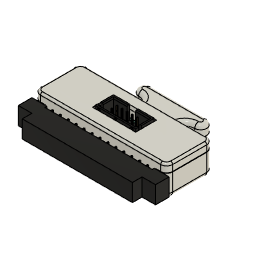
CBM8296_UP_Dongle v2 (Autodesk Fusion 360 design; units mm, degrees)
Autodesk Fusion 360 part; units mm, degrees
sketch "PCB" plane through (0, 0, 0) normal (0, 0, 1) x (1, 0, 0) in component "PCB"
  line L0 (54, 20) -> (0, 20)
  line L1 (0, 0) -> (54, 0)
  line L2 (54, 0) -> (54, 20)
  line L3 (0, 20) -> (0, 0)
  line L4 (1.3215, 4.5593) -> (1.3215, 2.9337)
  line L5 (2.4331, 2.9337) -> (3.3362, 2.9337)
  arc A0 (3.3362, 4.1529) -> (2.9298, 4.5593) centre (2.9298, 4.1529) ccw
  arc A1 (2.9298, 4.5593) -> (2.4331, 4.1981) centre (2.9298, 4.0372) ccw
  line L6 (0.87, 4.1981) -> (1.3215, 4.5593)
  line L7 (0.87, 2.9337) -> (1.7731, 2.9337)
  arc A2 (3.2007, 3.8368) -> (3.3362, 4.1529) centre (2.8997, 4.1529) ccw
  line L8 (3.2007, 3.8368) -> (2.4331, 2.9337)
  line L9 (43.09, -1) -> (43.09, 0)
  line L10 (46.55, 0) -> (46.55, -1)
  line L11 (51.01, -1) -> (51.01, 0)
  line L12 (51.01, 0) -> (50.51, 0)
  circle A3 centre (5, 15) radius 3.1789
  line L13 (50.51, 0) -> (50.51, -1)
  line L14 (45.82, 0.1) -> (45.82, -1)
  line L15 (43.09, 0) -> (42.59, 0)
  circle A4 centre (5, 15) radius 1.7463
  circle A5 centre (49, 15) radius 3.1789
  circle A6 centre (49, 15) radius 1.7463
  line L16 (49.78, 0.1) -> (49.78, -1)
  line L17 (43.82, 0.1) -> (43.82, -1)
  line L18 (7.45, -1) -> (7.45, 0)
  line L19 (3.49, 0) -> (2.99, 0)
  line L20 (37.9, 0.1) -> (37.9, -1)
  line L21 (24.02, 0.1) -> (24.02, -1)
  line L22 (34.67, 0) -> (34.67, -1)
  line L23 (22.79, 0) -> (22.79, -1)
  line L24 (23.29, 0) -> (22.79, 0)
  line L25 (29.98, 0.1) -> (29.98, -1)
  line L26 (38.63, 0) -> (38.63, -1)
  line L27 (35.17, -1) -> (35.17, 0)
  line L28 (27.25, 0) -> (26.75, 0)
  line L29 (26.75, 0) -> (26.75, -1)
  line L30 (35.17, 0) -> (34.67, 0)
  line L31 (47.05, -1) -> (47.05, 0)
  line L32 (33.94, 0.1) -> (33.94, -1)
  line L33 (23.29, -1) -> (23.29, 0)
  line L34 (47.05, 0) -> (46.55, 0)
  line L35 (27.98, 0.1) -> (27.98, -1)
  line L36 (42.59, 0) -> (42.59, -1)
  line L37 (41.86, 0.1) -> (41.86, -1)
  line L38 (35.9, 0.1) -> (35.9, -1)
  line L39 (30.71, 0) -> (30.71, -1)
  line L40 (27.25, -1) -> (27.25, 0)
  line L41 (31.94, 0.1) -> (31.94, -1)
  line L42 (39.86, 0.1) -> (39.86, -1)
  line L43 (26.02, 0.1) -> (26.02, -1)
  line L44 (39.13, 0) -> (38.63, 0)
  line L45 (47.78, 0.1) -> (47.78, -1)
  line L46 (31.21, 0) -> (30.71, 0)
  line L47 (10.18, 0.1) -> (10.18, -1)
  line L48 (7.45, 0) -> (6.95, 0)
  line L49 (8.18, 0.1) -> (8.18, -1)
  line L50 (6.22, 0.1) -> (6.22, -1)
  line L51 (4.22, 0.1) -> (4.22, -1)
  line L52 (3.49, -1) -> (3.49, 0)
  line L53 (39.13, -1) -> (39.13, 0)
  line L54 (31.21, -1) -> (31.21, 0)
  line L55 (53.8, -1) -> (0.2, -1)
  line L56 (6.95, 0) -> (6.95, -1)
  line L57 (0.2, -1) -> (0.2, 0)
  line L58 (0.2, 0) -> (-2.3, 0)
  line L59 (14.14, 0.1) -> (14.14, -1)
  line L60 (2.99, 0) -> (2.99, -1)
  line L61 (-7.25, 0) -> (-7.25, -6.8)
  line L62 (-2.3, 0) -> (-4, 0)
  line L63 (61.25, 0) -> (61.25, -6.8)
  line L64 (58, 0) -> (56.3, 0)
  line L65 (59.7, 0) -> (58, 0)
  line L66 (18.83, 0) -> (18.83, -1)
  line L67 (14.87, 0) -> (14.87, -1)
  line L68 (20.06, 0.1) -> (20.06, -1)
  line L69 (22.06, 0.1) -> (22.06, -1)
  line L70 (19.33, -1) -> (19.33, 0)
  line L71 (56.3, -1.6) -> (56.3, 0)
  line L72 (35.89, 15.3338) -> (35.89, 10.2537)
  line L73 (18.1, 0.1) -> (18.1, -1)
  line L74 (37.16, 8.825) -> (37.16, 7.3962)
  line L75 (16.84, 8.825) -> (16.84, 10.2537)
  line L76 (-4, 0) -> (-5.7, 0)
  line L77 (56.3, -6.8) -> (56.3, -5.2)
  line L78 (-2.3, -1.6) -> (-2.3, 0)
  line L79 (37.16, 7.3962) -> (16.84, 7.3962)
  line L80 (-5.7, -4.2) -> (-5.7, -2.6)
  line L81 (58, -7.2333) -> (58, -4.3667)
  line L82 (16.84, 7.3962) -> (16.84, 8.825)
  line L83 (16.1, 0.1) -> (16.1, -1)
  line L84 (-4, -8.7333) -> (-4, -11.6)
  line L85 (-5.7, -6.8) -> (-7.25, -6.8)
  line L86 (15.37, -1) -> (15.37, 0)
  line L87 (19.33, 0) -> (18.83, 0)
  line L88 (58, -8.052) -> (58, -7.9147)
  line L89 (-2.3, -4.2) -> (-2.3, -2.6)
  line L90 (-5.7, -6.8) -> (-5.7, -5.2)
  line L91 (18.11, 10.2537) -> (18.11, 15.3338)
  line L92 (12.14, 0.1) -> (12.14, -1)
  line L93 (59.7, -1.6) -> (59.7, 0)
  line L94 (15.37, 0) -> (14.87, 0)
  line L95 (29.0638, 16.6038) -> (37.16, 16.6038)
  line L96 (18.11, 15.3338) -> (24.9362, 15.3338)
  line L97 (16.84, 10.2537) -> (16.84, 16.6038)
  line L98 (-2.3, -6.8) -> (-2.3, -5.2)
  line L99 (10.91, 0) -> (10.91, -1)
  line L100 (24.9362, 16.6038) -> (29.0638, 16.6038)
  line L101 (11.41, -1) -> (11.41, 0)
  line L102 (24.9362, 15.3338) -> (29.0638, 15.3338)
  line L103 (56.3, -6.8) -> (54.5, -6.8)
  line L104 (11.41, 0) -> (10.91, 0)
  line L105 (-4, -4.3667) -> (-4, -7.2333)
  line L106 (59.7, -6.8) -> (59.7, -5.2)
  line L107 (37.16, 10.2537) -> (37.16, 8.825)
  line L108 (56.3, -4.2) -> (56.3, -2.6)
  line L109 (16.84, 16.6038) -> (24.9362, 16.6038)
  line L110 (-2.3, -6.8) -> (-5.7, -6.8)
  line L111 (54.5, -11.6) -> (-0.5, -11.6)
  line L112 (35.89, 8.6662) -> (18.11, 8.6662)
  line L113 (29.0638, 15.3338) -> (35.89, 15.3338)
  line L114 (35.89, 8.825) -> (35.89, 8.6662)
  line L115 (58, -2.8667) -> (58, 0)
  line L116 (-4, -3.548) -> (-4, -3.6853)
  line L117 (58, -3.6853) -> (58, -3.548)
  line L118 (-5.7, -1.6) -> (-5.7, 0)
  line L119 (17.6337, 10.2537) -> (16.84, 10.2537)
  line L120 (59.7, -4.2) -> (59.7, -2.6)
  line L121 (-4, -7.9147) -> (-4, -8.052)
  line L122 (58, -11.6) -> (58, -8.7333)
  line L123 (32.08, 14.6987) -> (32.3975, 15.0162)
  line L124 (61.25, 0) -> (59.7, 0)
  line L125 (36.3663, 8.19) -> (17.6337, 8.19)
  line L126 (36.3663, 8.19) -> (35.89, 8.6662)
  line L127 (35.89, 8.825) -> (36.3663, 8.825)
  line L128 (35.89, 10.2537) -> (36.3663, 10.2537)
  arc A7 (26.5238, 7.3962) -> (27.635, 7.3962) centre (27.0794, 7.3962) ccw
  line L129 (18.11, 8.6662) -> (17.6337, 8.19)
  line L130 (59.7, -6.8) -> (56.3, -6.8)
  line L131 (53.8, 0) -> (53.8, -1)
  line L132 (32.715, 15.0162) -> (32.5563, 15.0162)
  line L133 (32.5563, 15.0162) -> (32.3975, 15.0162)
  line L134 (31.9213, 15.0162) -> (32.08, 14.8575)
  line L135 (36.3663, 8.825) -> (37.16, 8.825)
  line L136 (36.3663, 8.19) -> (36.3663, 8.825)
  line L137 (24.9362, 15.3338) -> (24.9362, 15.81)
  line L138 (31.9213, 15.0162) -> (31.7625, 15.0162)
  line L139 (56.3, 0) -> (53.8, 0)
  line L140 (-4, 0) -> (-4, -2.8667)
  line L141 (24.9362, 15.81) -> (24.9362, 16.6038)
  line L142 (31.7625, 15.0162) -> (32.08, 14.6987)
  line L143 (18.11, 10.2537) -> (17.6337, 10.2537)
  line L144 (31.7625, 15.0162) -> (31.6038, 15.0162)
  line L145 (29.0638, 15.81) -> (36.3663, 15.81)
  line L146 (32.08, 14.54) -> (32.5563, 15.0162)
  line L147 (29.0638, 15.3338) -> (29.0638, 15.81)
  line L148 (18.11, 8.825) -> (18.11, 10.2537)
  line L149 (54.5, -6.8) -> (54.5, -11.6)
  line L150 (31.6038, 15.0162) -> (32.08, 14.54)
  line L151 (31.445, 15.0162) -> (32.08, 14.3812)
  line L152 (36.3663, 15.81) -> (35.89, 15.3338)
  line L153 (35.89, 10.2537) -> (35.89, 8.825)
  line L154 (-5.7, 0) -> (-7.25, 0)
  line L155 (18.11, 15.3338) -> (17.6337, 15.81)
  line L156 (-0.5, -11.6) -> (-0.5, -6.8)
  line L157 (17.6337, 8.825) -> (16.84, 8.825)
  arc A8 (18.11, 7.3962) -> (19.38, 7.3962) centre (18.745, 7.3962) ccw
  arc A9 (34.62, 7.3962) -> (35.89, 7.3962) centre (35.255, 7.3962) ccw
  line L158 (29.0638, 15.81) -> (29.0638, 16.6038)
  line L159 (-0.5, -6.8) -> (-2.3, -6.8)
  line L160 (32.08, 14.8575) -> (32.2388, 15.0162)
  line L161 (32.2388, 15.0162) -> (31.9213, 15.0162)
  line L162 (61.25, -6.8) -> (59.7, -6.8)
  line L163 (18.11, 8.6662) -> (18.11, 8.825)
  line L164 (37.16, 16.6038) -> (37.16, 10.2537)
  line L165 (31.6038, 15.0162) -> (31.445, 15.0162)
  line L166 (17.6337, 10.2537) -> (17.6337, 15.81)
  line L167 (32.08, 14.3812) -> (32.715, 15.0162)
  line L168 (32.3975, 15.0162) -> (32.2388, 15.0162)
  line L169 (36.3663, 10.2537) -> (36.3663, 15.81)
  line L170 (18.11, 8.825) -> (17.6337, 8.825)
  line L171 (36.3663, 10.2537) -> (37.16, 10.2537)
  line L172 (24.9362, 15.81) -> (17.6337, 15.81)
  line L173 (17.6337, 8.825) -> (17.6337, 8.19)
  line L174 (49.78, 0.1) -> (49.78, 4)
  line L175 (49.28, 3) -> (49.28, 2)
  arc A10 (44.32, 2) -> (45.32, 2) centre (44.82, 2) ccw
  line L176 (45.82, 0.1) -> (45.82, 4)
  line L177 (45.32, 3) -> (45.32, 2)
  arc A11 (45.32, 3) -> (44.32, 3) centre (44.82, 3) ccw
  arc A12 (49.78, 4) -> (47.78, 4) centre (48.78, 4) ccw
  arc A13 (49.28, 3) -> (48.28, 3) centre (48.78, 3) ccw
  line L178 (47.78, 0.1) -> (47.78, 4)
  arc A14 (45.82, 4) -> (43.82, 4) centre (44.82, 4) ccw
  line L179 (44.32, 3) -> (44.32, 2)
  line L180 (20.56, 3) -> (20.56, 2)
  arc A15 (17.6, 3) -> (16.6, 3) centre (17.1, 3) ccw
  line L181 (41.86, 0.1) -> (41.86, 4)
  arc A16 (33.44, 3) -> (32.44, 3) centre (32.94, 3) ccw
  line L182 (13.64, 3) -> (13.64, 2)
  arc A17 (6.22, 4) -> (4.22, 4) centre (5.22, 4) ccw
  line L183 (12.14, 0.1) -> (12.14, 4)
  arc A18 (5.72, 3) -> (4.72, 3) centre (5.22, 3) ccw
  arc A19 (26.02, 4) -> (24.02, 4) centre (25.02, 4) ccw
  arc A20 (36.4, 2) -> (37.4, 2) centre (36.9, 2) ccw
  arc A21 (48.28, 2) -> (49.28, 2) centre (48.78, 2) ccw
  arc A22 (24.52, 2) -> (25.52, 2) centre (25.02, 2) ccw
  line L184 (39.86, 0.1) -> (39.86, 4)
  arc A23 (28.48, 2) -> (29.48, 2) centre (28.98, 2) ccw
  arc A24 (16.6, 2) -> (17.6, 2) centre (17.1, 2) ccw
  arc A25 (10.18, 4) -> (8.18, 4) centre (9.18, 4) ccw
  line L185 (24.52, 3) -> (24.52, 2)
  arc A26 (18.1, 4) -> (16.1, 4) centre (17.1, 4) ccw
  arc A27 (13.64, 3) -> (12.64, 3) centre (13.14, 3) ccw
  arc A28 (9.68, 3) -> (8.68, 3) centre (9.18, 3) ccw
  arc A29 (33.94, 4) -> (31.94, 4) centre (32.94, 4) ccw
  arc A30 (41.86, 4) -> (39.86, 4) centre (40.86, 4) ccw
  line L186 (33.94, 0.1) -> (33.94, 4)
  arc A31 (20.56, 2) -> (21.56, 2) centre (21.06, 2) ccw
  line L187 (35.9, 0.1) -> (35.9, 4)
  line L188 (29.98, 0.1) -> (29.98, 4)
  line L189 (33.44, 3) -> (33.44, 2)
  line L190 (41.36, 3) -> (41.36, 2)
  arc A32 (4.72, 2) -> (5.72, 2) centre (5.22, 2) ccw
  line L191 (5.72, 3) -> (5.72, 2)
  line L192 (9.68, 3) -> (9.68, 2)
  line L193 (21.56, 3) -> (21.56, 2)
  line L194 (36.4, 3) -> (36.4, 2)
  line L195 (12.64, 3) -> (12.64, 2)
  line L196 (4.22, 0.1) -> (4.22, 4)
  line L197 (48.28, 3) -> (48.28, 2)
  arc A33 (8.68, 2) -> (9.68, 2) centre (9.18, 2) ccw
  line L198 (17.6, 3) -> (17.6, 2)
  arc A34 (22.06, 4) -> (20.06, 4) centre (21.06, 4) ccw
  arc A35 (41.36, 3) -> (40.36, 3) centre (40.86, 3) ccw
  line L199 (37.9, 0.1) -> (37.9, 4)
  line L200 (32.44, 3) -> (32.44, 2)
  line L201 (31.94, 0.1) -> (31.94, 4)
  line L202 (4.72, 3) -> (4.72, 2)
  arc A36 (37.4, 3) -> (36.4, 3) centre (36.9, 3) ccw
  arc A37 (29.48, 3) -> (28.48, 3) centre (28.98, 3) ccw
  line L203 (16.6, 3) -> (16.6, 2)
  line L204 (20.06, 0.1) -> (20.06, 4)
  arc A38 (40.36, 2) -> (41.36, 2) centre (40.86, 2) ccw
  line L205 (27.98, 0.1) -> (27.98, 4)
  line L206 (26.02, 0.1) -> (26.02, 4)
  line L207 (24.02, 0.1) -> (24.02, 4)
  line L208 (28.48, 3) -> (28.48, 2)
  arc A39 (29.98, 4) -> (27.98, 4) centre (28.98, 4) ccw
  arc A40 (37.9, 4) -> (35.9, 4) centre (36.9, 4) ccw
  line L209 (29.48, 3) -> (29.48, 2)
  line L210 (6.22, 0.1) -> (6.22, 4)
  line L211 (43.82, 0.1) -> (43.82, 4)
  arc A41 (25.52, 3) -> (24.52, 3) centre (25.02, 3) ccw
  arc A42 (32.44, 2) -> (33.44, 2) centre (32.94, 2) ccw
  line L212 (25.52, 3) -> (25.52, 2)
  line L213 (22.06, 0.1) -> (22.06, 4)
  line L214 (37.4, 3) -> (37.4, 2)
  line L215 (40.36, 3) -> (40.36, 2)
  line L216 (24.206, 13.016) -> (24.714, 13.016)
  line L217 (31.826, 10.984) -> (31.826, 10.476)
  line L218 (31.826, 10.476) -> (32.334, 10.476)
  line L219 (31.826, 13.016) -> (32.334, 13.016)
  line L220 (32.334, 13.016) -> (32.334, 13.524)
  line L221 (24.714, 13.524) -> (24.206, 13.524)
  line L222 (29.286, 10.476) -> (29.794, 10.476)
  line L223 (29.286, 13.524) -> (29.286, 13.016)
  line L224 (31.826, 13.524) -> (31.826, 13.016)
  line L225 (24.206, 10.984) -> (24.206, 10.476)
  line L226 (26.746, 10.476) -> (27.254, 10.476)
  line L227 (26.746, 13.524) -> (26.746, 13.016)
  line L228 (29.794, 10.984) -> (29.286, 10.984)
  line L229 (14.14, 0.1) -> (14.14, 4)
  line L230 (21.666, 13.016) -> (22.174, 13.016)
  line L231 (21.666, 13.524) -> (21.666, 13.016)
  line L232 (21.666, 10.476) -> (22.174, 10.476)
  line L233 (8.18, 0.1) -> (8.18, 4)
  line L234 (22.174, 13.016) -> (22.174, 13.524)
  line L235 (27.254, 10.476) -> (27.254, 10.984)
  line L236 (29.794, 13.524) -> (29.286, 13.524)
  line L237 (24.714, 10.984) -> (24.206, 10.984)
  line L238 (24.206, 13.524) -> (24.206, 13.016)
  line L239 (29.794, 13.016) -> (29.794, 13.524)
  line L240 (10.18, 0.1) -> (10.18, 4)
  line L241 (16.1, 0.1) -> (16.1, 4)
  line L242 (32.334, 10.984) -> (31.826, 10.984)
  line L243 (29.286, 10.984) -> (29.286, 10.476)
  arc A43 (12.64, 2) -> (13.64, 2) centre (13.14, 2) ccw
  line L244 (29.794, 10.476) -> (29.794, 10.984)
  line L245 (29.286, 13.016) -> (29.794, 13.016)
  line L246 (8.68, 3) -> (8.68, 2)
  line L247 (32.334, 13.524) -> (31.826, 13.524)
  line L248 (24.714, 13.016) -> (24.714, 13.524)
  arc A44 (14.14, 4) -> (12.14, 4) centre (13.14, 4) ccw
  line L249 (27.254, 10.984) -> (26.746, 10.984)
  line L250 (24.206, 10.476) -> (24.714, 10.476)
  line L251 (18.1, 0.1) -> (18.1, 4)
  line L252 (44, 12.25) -> (44, 12.2)
  line L253 (26.746, 13.016) -> (27.254, 13.016)
  line L254 (22.174, 10.984) -> (21.666, 10.984)
  line L255 (21.666, 10.984) -> (21.666, 10.476)
  line L256 (26.746, 10.984) -> (26.746, 10.476)
  line L257 (22.174, 10.476) -> (22.174, 10.984)
  line L258 (24.714, 10.476) -> (24.714, 10.984)
  line L259 (27.254, 13.524) -> (26.746, 13.524)
  line L260 (32.334, 10.476) -> (32.334, 10.984)
  arc A45 (21.56, 3) -> (20.56, 3) centre (21.06, 3) ccw
  line L261 (27.254, 13.016) -> (27.254, 13.524)
  line L262 (22.174, 13.524) -> (21.666, 13.524)
extrude "Extrude1" add sketch "PCB" against normal blind 1.6 contours L0 L1 L2 L3 L12 L14 L15 L16 L17 L19 L20 L21 L24 L25 L28 L30 L32 L34 L35 L37 L38 L41 L42 L43 L44 L45 L46 L47 L48 L49 L50 L51 L58 L59 L68 L69 L73 L83 L87 L92 L94 L104 L139 L174 L176 A12 L178 A14 L181 A17 L183 A19 L184 A25 A26 A29 A30 L186 L187 L188 L196 A34 L199 L201 L204 L205 L206 L207 A39 A40 L210 L211 L213 L229 L233 L240 L241 A44 L251 | L1 L16 L45 L174 A12 L178 | L1 L50 L51 A17 L196 L210 | L1 L14 L17 L176 A14 L211 | L1 L47 L49 A25 L233 L240 | L1 L37 L42 L181 L184 A30 | L1 L59 L92 L183 L229 A44 | L1 L20 L38 L187 L199 A40 | L1 L73 L83 A26 L241 L251 | L1 L32 L41 A29 L186 L201 | L1 L68 L69 A34 L204 L213 | L1 L25 L35 L188 L205 A39 | L1 L21 L43 A19 L206 L207 | A3 | A5 | L72 L128 L152 L169 | L72 L91 L96 L102 L112 L113 L114 L148 L153 L163 | L113 L145 L147 L152 | L107 L127 L128 L135 L153 L171 | L100 L102 L137 L141 L147 L158 | L95 L145 L158 L164 L169 L171 | L114 L126 L127 L136 | L96 L137 L155 L172 | L112 L125 L126 L129 | L74 L79 L82 L125 L135 L136 L157 L173 | L91 L143 L155 L166 | L97 L109 L119 L141 L166 L172 | L129 L163 L170 L173 | L75 L119 L143 L148 L157 L170 | L79 A9 | L79 A7 | L79 A8 | L123 L134 L138 L142 L160 L168 | L123 L133 L142 L144 L146 L150 | L132 L146 L150 L151 L165 L167 | L134 L160 L161 | L175 A13 A21 L197 | A10 L177 A11 L179 | L180 A31 L193 A45 | A15 A24 L198 L203 | A16 L189 L200 A42 | L182 A27 L195 A43 | A18 A32 L191 L202 | A20 L194 A36 L214 | A22 L185 A41 L212 | A23 A37 L208 L209 | A28 L192 A33 L246 | L190 A35 A38 L215 | L216 L221 L238 L248 | L217 L218 L242 L260 | L219 L220 L224 L247 | L222 L228 L243 L244 | L223 L236 L239 L245 | L225 L237 L250 L258 | L226 L235 L249 L256 | L227 L253 L259 L261 | L230 L231 L234 L262 | L232 L254 L255 L257 makes body 1 in component "PCB"
extrude "Extrude5" add sketch "PCB" along normal blind 2.3 contours L72 L91 L96 L102 L112 L113 L114 L148 L153 L163 | L107 L127 L128 L135 L153 L171 | L100 L102 L137 L141 L147 L158 | L75 L119 L143 L148 L157 L170 bodies 1 in component "PCB"
extrude "Extrude6" add sketch "PCB" along normal blind 9.3 contours L72 L128 L152 L169 | L113 L145 L147 L152 | L95 L145 L158 L164 L169 L171 | L114 L126 L127 L136 | L96 L137 L155 L172 | L112 L125 L126 L129 | L74 L79 L82 L125 L135 L136 L157 L173 | L91 L143 L155 L166 | L97 L109 L119 L141 L166 L172 | L129 L163 L170 L173 bodies 1 in component "PCB"
extrude "Extrude7" add sketch "PCB" along normal blind 8.8 contours L216 L221 L238 L248 | L217 L218 L242 L260 | L219 L220 L224 L247 | L222 L228 L243 L244 | L223 L236 L239 L245 | L225 L237 L250 L258 | L226 L235 L249 L256 | L227 L253 L259 L261 | L230 L231 L234 L262 | L232 L254 L255 L257 bodies 1 in component "PCB"
extrude "Extrude8" add sketch "PCB" along normal blind 8.8 contours L79 A9 | L79 A7 | L79 A8 bodies 1 in component "PCB"
extrude "Extrude9" add sketch "PCB" along normal blind 4.3 and the other way blind 4.4 contours L1 L55 L57 L58 L61 L62 L63 L64 L65 L76 L85 L103 L110 L111 L124 L130 L131 L139 L149 L154 L156 L159 L162 | L1 L11 L12 L13 L55 | L1 L19 L52 L55 L60 | L1 L10 L31 L34 L55 | L1 L18 L48 L55 L56 | L1 L9 L15 L36 L55 | L1 L55 L99 L101 L104 | L1 L26 L44 L53 L55 | L1 L55 L67 L86 L94 | L1 L22 L27 L30 L55 | L1 L55 L66 L70 L87 | L1 L39 L46 L54 L55 | L1 L23 L24 L33 L55 | L1 L28 L29 L40 L55 bodies 1 in component "PCB"
extrude "Extrude10" add sketch "PCB" along normal blind 0.5 contours L1 L16 L45 L55 | L1 L16 L45 L174 A12 L178 | L1 L50 L51 A17 L196 L210 | L1 L50 L51 L55 | L1 L14 L17 L55 | L1 L14 L17 L176 A14 L211 | L1 L47 L49 A25 L233 L240 | L1 L47 L49 L55 | L1 L37 L42 L55 | L1 L37 L42 L181 L184 A30 | L1 L59 L92 L183 L229 A44 | L1 L55 L59 L92 | L1 L20 L38 L55 | L1 L20 L38 L187 L199 A40 | L1 L73 L83 A26 L241 L251 | L1 L55 L73 L83 | L1 L32 L41 L55 | L1 L32 L41 A29 L186 L201 | L1 L68 L69 A34 L204 L213 | L1 L55 L68 L69 | L1 L25 L35 L55 | L1 L25 L35 L188 L205 A39 | L1 L21 L43 A19 L206 L207 | L1 L21 L43 L55 bodies 1 in component "PCB"
extrude "Extrude11" add sketch "PCB" against normal blind 0.5 from surface at -1.6 contours L1 L16 L45 L55 | L1 L16 L45 L174 A12 L178 | L1 L50 L51 A17 L196 L210 | L1 L50 L51 L55 | L1 L14 L17 L55 | L1 L14 L17 L176 A14 L211 | L1 L47 L49 A25 L233 L240 | L1 L47 L49 L55 | L1 L37 L42 L55 | L1 L37 L42 L181 L184 A30 | L1 L59 L92 L183 L229 A44 | L1 L55 L59 L92 | L1 L20 L38 L55 | L1 L20 L38 L187 L199 A40 | L1 L73 L83 A26 L241 L251 | L1 L55 L73 L83 | L1 L32 L41 L55 | L1 L32 L41 A29 L186 L201 | L1 L68 L69 A34 L204 L213 | L1 L55 L68 L69 | L1 L25 L35 L55 | L1 L25 L35 L188 L205 A39 | L1 L21 L43 A19 L206 L207 | L1 L21 L43 L55 bodies 1 in component "PCB"
chamfer "Chamfer1" distance 0.5 angle 45 7 edges at (27, 8.6662, 9.3) (35.89, 12.7938, 9.3) (32.4769, 15.3338, 9.3) (21.5231, 15.3338, 9.3) (18.11, 12.7938, 9.3) (18.11, 8.7456, 9.3) (35.89, 8.7456, 9.3) on bodies 1 in component "PCB"
ref_plane "WorkPlane1" through (0, 0, -4.4) normal (0, 0, 1) x (1, 0, 0) in component "bottom_shell"
sketch "bottom" plane through (0, 0, -4.4) normal (0, 0, 1) x (1, 0, 0) in component "bottom_shell"
  circle A0 centre (49, 15) radius 1.7463 construction
  line L0 (54, 0) -> (54, 20) construction
  line L1 (54, 20) -> (0, 20) construction
  line L2 (0, 20) -> (0, 0) construction
  circle A1 centre (5, 15) radius 1.7463 construction
  line L3 (27, 20) -> (27, -5) construction
  line L4 (54, 0) -> (0, 0) construction
  circle A2 centre (49, 15) radius 1.75
  circle A3 centre (5, 15) radius 1.75
  line L5 (60, 3) -> (60, 20)
  line L6 (-6, 3) -> (-6, 20)
  line L7 (57, 23) -> (-3, 23)
  line L8 (57, 0) -> (-3, 0)
  arc A4 (57, 0) -> (60, 3) centre (57, 3) ccw
  arc A5 (60, 20) -> (57, 23) centre (57, 20) ccw
  arc A6 (-3, 23) -> (-6, 20) centre (-3, 20) ccw
  arc A7 (-6, 3) -> (-3, 0) centre (-3, 3) ccw
  line L9 (57, 21) -> (-3, 21)
  arc A8 (-3, 21) -> (-4, 20) centre (-3, 20) ccw
  line L10 (-4, 3) -> (-4, 20)
  arc A9 (-4, 3) -> (-3, 2) centre (-3, 3) ccw
  line L11 (57, 2) -> (-3, 2)
  arc A10 (57, 2) -> (58, 3) centre (57, 3) ccw
  line L12 (58, 3) -> (58, 20)
  arc A11 (58, 20) -> (57, 21) centre (57, 20) ccw
  circle A12 centre (49, 15) radius 4.25
  circle A13 centre (5, 15) radius 4.25
  line L13 (54.6, 1.2) -> (54.6, 2)
  line L14 (-0.6, 0) -> (-0.6, 2)
  circle A14 centre (49, 15) radius 3
  circle A15 centre (5, 15) radius 3
  line L15 (57, 21.8) -> (-3, 21.8)
  arc A16 (-3, 21.8) -> (-4.8, 20) centre (-3, 20) ccw
  line L16 (-4.8, 3) -> (-4.8, 20)
  arc A17 (-4.8, 3) -> (-3, 1.2) centre (-3, 3) ccw
  arc A18 (57, 1.2) -> (58.8, 3) centre (57, 3) ccw
  line L17 (58.8, 3) -> (58.8, 20)
  arc A19 (58.8, 20) -> (57, 21.8) centre (57, 20) ccw
  line L18 (57, 1.2) -> (54.6, 1.2)
  line L19 (-0.6, 1.2) -> (-3, 1.2)
  line L20 (54.6, 1.2) -> (54.6, 0)
  line L21 (41, 28) -> (41, 33) construction
  line L22 (41, 33) -> (13, 33) construction
  line L23 (41, 33) -> (41, 39.5) construction
  line L24 (13, 39) -> (41, 39)
  line L25 (13, 36) -> (13, 39) construction
  arc A20 (13, 39) -> (13, 33) centre (13, 36) ccw
  arc A21 (41, 33) -> (41, 39) centre (41, 36) ccw
  arc A22 (41, 33) -> (41, 23) centre (41, 28) ccw
  arc A23 (13, 23) -> (13, 33) centre (13, 28) ccw
  point P0 (51.01, 0)
  point P1 (60, 0)
  point P2 (60, 23)
  point P3 (-6, 0)
  point P4 (-6, 23)
  dimension "d181" = 3.5
  dimension "d182" = 3.5
  dimension "d186" = 3
  dimension "d187" = 23
  dimension "d188" = 66
  dimension "d190" = 8.5
  dimension "d191" = 8.5
  dimension "d192" = 0.6
  dimension "d193" = 0.6
  dimension "d194" = 6
  dimension "d195" = 6
  dimension "d197" = 1.2
  dimension "d236" = 10
  dimension "d237" = 14
  dimension "d238" = 5
  dimension "d239" = 6
  constraint midpoint L1 L3.start
  constraint perpendicular L1 L3
  constraint coincident L0.start L4.start
  constraint coincident L2.end L4.end
  constraint concentric A0 A2
  constraint concentric A1 A3
  constraint vertical L5
  constraint perpendicular L4 L6
  constraint symmetric L3 L5 L6
  constraint perpendicular L5 L7
  constraint collinear L4 L8
  constraint coincident P1 L5
  constraint tangent L5 A4
  constraint tangent L8 A4
  constraint coincident P2 L5
  constraint coincident P2 L7
  constraint tangent L5 A5
  constraint tangent L7 A5
  constraint equal A4 A5
  constraint coincident P4 L6
  constraint coincident P4 L7
  constraint tangent L6 A6
  constraint tangent L7 A6
  constraint equal A4 A6
  constraint coincident P3 L6
  constraint coincident P3 L8
  constraint tangent L6 A7
  constraint tangent L8 A7
  constraint equal A4 A7
  constraint concentric A0 A12
  constraint concentric A3 A13
  constraint coincident L11 L13.end
  constraint perpendicular L11 L13
  constraint coincident L8 L14.start
  constraint coincident L11 L14.end
  constraint perpendicular L11 L14
  constraint concentric A2 A14
  constraint concentric A3 A15
  constraint parallel L7 L15
  constraint concentric A6 A16
  constraint parallel L6 L16
  constraint concentric A7 A17
  constraint parallel L8 L18
  constraint concentric A4 A18
  constraint parallel L5 L17
  constraint concentric A5 A19
  constraint tangent L15 A19
  constraint tangent A16 L16
  constraint tangent L15 A16
  constraint tangent L17 A19
  constraint tangent L16 A17
  constraint tangent A17 L18
  constraint tangent A18 L18
  constraint tangent A18 L17
  constraint collinear L18 L19
  constraint coincident L14 L19.start
  constraint coincident L8 L20.end
  constraint perpendicular L8 L20
  constraint symmetric L3 A22 A23
  constraint coincident L21.start A22.centre
  constraint vertical L21
  constraint tangent L22 A23
  constraint tangent L22 A21
  constraint perpendicular L22 L23
  constraint coincident A21.centre L23
  constraint symmetric L3 A20 A21
  constraint coincident L23 L24.end
  constraint tangent L24 A21
  constraint coincident L25.start A20.centre
  constraint perpendicular L24 L25
  constraint coincident L7 A22.end
  constraint coincident L7 A23.start
  measures "d181" diameter of A2
  measures "d182" diameter of A3
  measures "d186" radius of A4
  measures "d187" distance of L7 L8
  measures "d188" distance of L5 L6
  measures "d190" diameter of A12
  measures "d191" diameter of A13
  measures "d192" distance of L0 L13
  measures "d193" distance of L2 L14
  measures "d194" diameter of A14
  measures "d195" diameter of A15
  measures "d197" distance of L7 L15
  measures "d236" diameter of A22
  measures "d237" distance of L3 L21.start
  measures "d238" distance of L7 L21.start
  measures "d239" diameter of A21
extrude "Extrude1'" add sketch "bottom" against normal blind 2 separate body contours L5 L6 L7 L8 A4 A5 A6 A7 L14 L15 A16 L16 A17 A18 L17 A19 L18 L19 L20 | L8 L11 L13 L14 L20 | L7 L24 A20 A21 A22 A23 | L9 A8 L10 A9 L11 A10 L12 A11 L13 L14 L15 A16 L16 A17 A18 L17 A19 L18 L19 | L9 A8 L10 A9 L11 A10 L12 A11 | A12 | A13 makes body 2 in component "bottom_shell"
extrude "Extrude2" add sketch "bottom" along normal blind 2.8 contours A12 | A13 | A14 | A15 bodies 2 in component "bottom_shell"
extrude "Extrude3" add sketch "bottom" along normal blind 1.8 contours L8 L11 L13 L14 L20 bodies 2 in component "bottom_shell"
extrude "Extrude4" add sketch "bottom" along normal blind 9.7 contours L9 A8 L10 A9 L11 A10 L12 A11 L13 L14 L15 A16 L16 A17 A18 L17 A19 L18 L19 bodies 2 in component "bottom_shell"
extrude "Extrude5'" add sketch "bottom" along normal blind 8.7 contours L5 L6 L7 L8 A4 A5 A6 A7 L14 L15 A16 L16 A17 A18 L17 A19 L18 L19 L20 bodies 2 in component "bottom_shell"
extrude "Extrude6'" add sketch "bottom" along normal blind 5 contours L7 L24 A20 A21 A22 A23 bodies 2 in component "bottom_shell"
fillet "Fillet1" radius 1 8 edges at (27, 2, -4.4) (57.7071, 2.2929, -4.4) (58, 11.5, -4.4) (57.7071, 20.7071, -4.4) (27, 21, -4.4) (-3.7071, 20.7071, -4.4) (-4, 11.5, -4.4) (-3.7071, 2.2929, -4.4) on bodies 2 in component "bottom_shell"
fillet "Fillet2" radius 1 2 edges at (1.0376, 16.5369, -4.4) (45.0376, 16.5369, -4.4) on bodies 2 in component "bottom_shell"
chamfer "Chamfer1'" distance 1 angle 45 2 edges at (1.0376, 13.4631, -1.6) (45.0376, 13.4631, -1.6) on bodies 2 in component "bottom_shell"
fillet "Fillet4" radius 2 20 edges at (5, 23, -6.4) (18, 28, -6.4) (10, 36, -6.4) (27, 39, -6.4) (44, 36, -6.4) (36, 28, -6.4) (49, 23, -6.4) (59.1213, 22.1213, -6.4) (60, 11.5, -6.4) (59.1213, 0.8787, -6.4) (27, 0, -6.4) (-5.1213, 0.8787, -6.4) (-6, 11.5, -6.4) (-5.1213, 22.1213, -6.4) (36, 28, 0.6) (44, 36, 0.6) (27, 39, 0.6) (10, 36, 0.6) (18, 28, 0.6) (27, 23, 0.6) on bodies 2 in component "bottom_shell"
ref_plane "WorkPlane1" through (0, 0, 6.5) normal (0, 0, 1) x (1, 0, 0) in component "top_shell"
sketch "top" plane through (0, 0, 6.5) normal (0, 0, 1) x (1, 0, 0) in component "top_shell"
  line L0 (16.84, 16.6038) -> (24.9362, 16.6038) construction
  line L1 (24.9362, 16.6038) -> (29.0638, 16.6038) construction
  line L2 (16.84, 10.2537) -> (16.84, 16.6038) construction
  line L3 (16.84, 8.825) -> (16.84, 10.2537) construction
  line L4 (16.84, 7.3962) -> (16.84, 8.825) construction
  line L5 (37.16, 7.3962) -> (16.84, 7.3962) construction
  line L6 (37.16, 8.825) -> (37.16, 7.3962) construction
  line L7 (37.16, 10.2537) -> (37.16, 8.825) construction
  line L8 (37.16, 16.6038) -> (37.16, 10.2537) construction
  line L9 (29.0638, 16.6038) -> (37.16, 16.6038) construction
  line L10 (57, 23) -> (-3, 23)
  arc A0 (-3, 23) -> (-6, 20) centre (-3, 20) ccw
  line L11 (-6, 3) -> (-6, 20)
  arc A1 (-6, 3) -> (-3, 0) centre (-3, 3) ccw
  line L12 (57, 0) -> (-3, 0)
  line L13 (57, 2) -> (-3, 2)
  arc A2 (-4, 3) -> (-3, 2) centre (-3, 3) ccw
  line L14 (-4, 3) -> (-4, 20)
  arc A3 (-3, 21) -> (-4, 20) centre (-3, 20) ccw
  line L15 (57, 21) -> (-3, 21)
  line L16 (58, 3) -> (58, 20)
  arc A4 (58, 20) -> (57, 21) centre (57, 20) ccw
  arc A5 (57, 2) -> (58, 3) centre (57, 3) ccw
  arc A6 (57, 0) -> (60, 3) centre (57, 3) ccw
  line L17 (60, 3) -> (60, 20)
  arc A7 (60, 20) -> (57, 23) centre (57, 20) ccw
  line L18 (-0.6, 0) -> (-0.6, 2)
  line L19 (54.6, 1.2) -> (54.6, 0)
  line L20 (54.6, 1.2) -> (54.6, 2)
  circle A8 centre (5, 15) radius 1.75 construction
  circle A9 centre (49, 15) radius 1.75 construction
  circle A10 centre (5, 15) radius 1.25
  circle A11 centre (49, 15) radius 1.25
  line L21 (16.24, 17.2038) -> (37.76, 17.2038)
  line L22 (37.76, 17.2038) -> (37.76, 6.7962)
  line L23 (37.76, 6.7962) -> (16.24, 6.7962)
  line L24 (16.24, 6.7962) -> (16.24, 17.2038)
  circle A12 centre (5, 15) radius 3.5
  circle A13 centre (49, 15) radius 3.5
  line L25 (59.2, 3) -> (59.2, 20)
  arc A14 (59.2, 20) -> (57, 22.2) centre (57, 20) ccw
  line L26 (57, 22.2) -> (-3, 22.2)
  arc A15 (-3, 22.2) -> (-5.2, 20) centre (-3, 20) ccw
  line L27 (-5.2, 3) -> (-5.2, 20)
  arc A16 (-5.2, 3) -> (-3, 0.8) centre (-3, 3) ccw
  arc A17 (57, 0.8) -> (59.2, 3) centre (57, 3) ccw
  line L28 (57, 0.8) -> (54.6, 0.8)
  line L29 (-0.6, 0.8) -> (-3, 0.8)
  dimension "d213" = 2.5
  dimension "d214" = 2.5
  dimension "d216" = 0.6
  dimension "d217" = 0.6
  dimension "d218" = 0.6
  dimension "d219" = 0.6
  dimension "d220" = 7
  dimension "d221" = 7
  dimension "d223" = 0.8
  constraint concentric A8 A10
  constraint concentric A9 A11
  constraint horizontal L21
  constraint vertical L22
  constraint horizontal L23
  constraint vertical L24
  constraint concentric A10 A12
  constraint concentric A11 A13
  constraint parallel L17 L25
  constraint concentric A7 A14
  constraint parallel L10 L26
  constraint concentric A0 A15
  constraint parallel L11 L27
  constraint concentric A1 A16
  constraint parallel L12 L28
  constraint concentric A6 A17
  constraint tangent L27 A16
  constraint tangent L25 A17
  constraint tangent A16 L28
  constraint tangent L25 A14
  constraint tangent A14 L26
  constraint tangent L26 A15
  constraint tangent A15 L27
  constraint tangent A17 L28
  constraint coincident L19 L28.end
  constraint coincident L18 L29.start
  constraint collinear L28 L29
  measures "d213" diameter of A10
  measures "d214" diameter of A11
  measures "d216" distance of L0 L21
  measures "d217" distance of L5 L23
  measures "d218" distance of L2 L24
  measures "d219" distance of L6 L22
  measures "d220" diameter of A12
  measures "d221" diameter of A13
  measures "d223" distance of L10 L26
extrude "Extrude1''" add sketch "top" along normal blind 2 separate body contours L10 A0 L11 A1 L12 A6 L17 A7 L18 L19 L25 A14 L26 A15 L27 A16 A17 L28 L29 | L12 L13 L18 L19 L20 | L13 A2 L14 A3 L15 L16 A4 A5 L18 L19 L20 L25 A14 L26 A15 L27 A16 A17 L28 L29 | L13 A2 L14 A3 L15 L16 A4 A5 | A10 | A11 | A12 | A13 makes body 3 in component "top_shell"
extrude "Extrude2'" add sketch "top" against normal blind 6.3 contours A12 | A13 bodies 3 in component "top_shell"
extrude "Extrude3'" add sketch "top" against normal blind 1 contours L13 A2 L14 A3 L15 L16 A4 A5 L18 L19 L20 L25 A14 L26 A15 L27 A16 A17 L28 L29 bodies 3 in component "top_shell"
extrude "Extrude4'" add sketch "top" against normal blind 3.5 contours L12 L13 L18 L19 L20 bodies 3 in component "top_shell"
extrude "Extrude5''" add sketch "top" against normal blind 2 contours L10 A0 L11 A1 L12 A6 L17 A7 L18 L19 L25 A14 L26 A15 L27 A16 A17 L28 L29 bodies 3 in component "top_shell"
fillet "Fillet1'" radius 1 10 edges at (27, 21, 6.5) (57.7071, 20.7071, 6.5) (58, 11.5, 6.5) (57.7071, 2.2929, 6.5) (27, 2, 6.5) (-3.7071, 2.2929, 6.5) (-4, 11.5, 6.5) (-3.7071, 20.7071, 6.5) (1.7369, 13.7343, 6.5) (45.7369, 13.7343, 6.5) on bodies 3 in component "top_shell"
fillet "Fillet2'" radius 1 8 edges at (-6, 11.5, 8.5) (-5.1213, 0.8787, 8.5) (27, 0, 8.5) (59.1213, 0.8787, 8.5) (60, 11.5, 8.5) (59.1213, 22.1213, 8.5) (27, 23, 8.5) (-5.1213, 22.1213, 8.5) on bodies 3 in component "top_shell"
component "PCB" placed x (1, 0, 0) y (0, 1, 0) z (0, 0, 1) at (0, 0, 0)
component "bottom_shell" placed x (1, 0, 0) y (0, 1, 0) z (0, 0, 1) at (0, 0, 0)
component "top_shell" placed x (1, 0, 0) y (0, 1, 0) z (0, 0, 1) at (0, 0, 0)
equation "pcb_thickness = 1.6 mm"
equation "below = 2.8 mm + pcb_thickness"
equation "wall = 2 mm"
equation "width = pcb_width + 2 mm + 2 * r_corner + 2 * wall"
equation "length = pcb_length + 1 mm + wall"
equation "above = 8.5 mm - wall"
equation "pcb_width = 54 mm"
equation "pcb_length = 20 mm"
equation "r_corner = 3 mm"
equation "drill = 3.5 mm"
equation "d_screw = 7 mm"
equation "tol_x = 0.3 mm"
equation "tol_connector = 0.6 mm"
equation "d_post = 8.5 mm"
equation "d_post2 = 8 mm"
equation "bottom_height = 4.3 mm + below"
equation "overlap = 1 mm"
equation "top_height = above + below - bottom_height - tol_y"
equation "d35 = tol_connector"
equation "d37 = d35"
equation "tol_y = 0.2 mm"
equation "d154 = -pcb_thickness"
equation "d176 = -pcb_thickness"
equation "d180 = -below"
equation "d181 = drill"
equation "d182 = drill"
equation "d186 = r_corner"
equation "d187 = length"
equation "d188 = width"
equation "d189 = -wall"
equation "d190 = d_post"
equation "d191 = d_post"
equation "d192 = tol_connector"
equation "d193 = tol_connector"
equation "d195 = d194"
equation "d197 = 0.6 * wall"
equation "d198 = -wall"
equation "d200 = below - pcb_thickness"
equation "d202 = below - pcb_thickness - 1 mm"
equation "d204 = bottom_height + overlap"
equation "d206 = bottom_height"
equation "d212 = above"
equation "d216 = tol_connector"
equation "d217 = tol_connector"
equation "d218 = tol_connector"
equation "d219 = tol_connector"
equation "d220 = d_screw"
equation "d221 = d_screw"
equation "d223 = 0.4 * wall"
equation "d224 = wall"
equation "d226 = -above + tol_y"
equation "d228 = -top_height + overlap"
equation "d230 = -top_height - 1.5 mm"
equation "d232 = -top_height"
equation "d238 = d236 / 2"
named bodies: "PCB", "bottom", "top"
